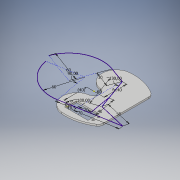
# Autodesk Inventor part: wstepna_geometria_wersja_2
Saved by Autodesk Inventor 2019 (Build 230136000, 136)
## iProperties
Created: 2022-02-09
Part Number: wstepna_geometria_wersja_2
Material: Generic
Document SubType Name: Modeling
Designer: Tomasz Krakowski
Density: 1 g/cm^3
Appearance: Default
Author: Tomasz Krakowski
Autodesk Inventor part; units mm, degrees
ref_plane "YZ Plane" through (0, 0, 0) normal (1, 0, 0) x (0, 1, 0)
ref_plane "XZ Plane" through (0, 0, 0) normal (0, 1, 0) x (-1, 0, 0)
ref_plane "XY Plane" through (0, 0, 0) normal (0, 0, 1) x (1, 0, 0)
sketch "Sketch1" plane through (0, 0, 0) normal (0, 1, 0) x (-1, 0, 0)
  arc A0 (-1.4142, 9.8995) -> (-10, 0) centre (0, 0) ccw
  line L0 (-39.5, 50) -> (0.5, 50)
  line L1 (0.5, 50) -> (0.5, 30)
  line L2 (0.5, 30) -> (-39.5, 30)
  line L3 (-39.5, 30) -> (-39.5, 50)
  line L4 (-39.5, 50) -> (0.5, 30) construction
  line L5 (0.5, 50) -> (-39.5, 30) construction
  line L6 (-10, 40) -> (-19.5, 40) construction
  circle A1 centre (4.5, 35.25) radius 1.9
  circle A2 centre (4.5, 44.75) radius 1.9
  line L7 (4.5, 44.75) -> (4.5, 35.25) construction
  circle A3 centre (-43.5, 44.75) radius 1.9
  circle A4 centre (-43.5, 35.25) radius 1.9
  line L8 (-43.5, 44.75) -> (-43.5, 35.25) construction
  line L9 (-43.5, 40) -> (-19.5, 40) construction
  line L10 (-10, 40) -> (4.5, 40) construction
  line L11 (-43.5, 44.75) -> (4.5, 44.75) construction
  line L12 (-43.5, 35.25) -> (4.5, 35.25) construction
  line L13 (-19.5, 40) -> (-19.5, 44.75) construction
  circle A5 centre (-10, 40) radius 9.75 construction
  circle A6 centre (-29, 40) radius 9.75 construction
  arc A7 (-2.7044, 60.2512) -> (-52.4397, 48.5007) centre (-10, -20) ccw
  arc A8 (-1.4142, 9.8995) -> (-2.7044, 60.2512) centre (-5, 35) ccw
  line L14 (-57.1731, 40) -> (-57.1731, 0)
  line L15 (-57.1731, 0) -> (0, 0) construction
  arc A9 (-52.4397, 48.5007) -> (-57.1731, 40) centre (-47.1731, 40) ccw
  line L16 (0, 0) -> (10, 0) construction
  line L17 (-10, 0) -> (-57.1731, 0) construction
  arc A10 (-10, 0) -> (-1.4142, -9.8995) centre (0, 0) ccw
  arc A11 (-52.4397, -48.5007) -> (-2.7044, -60.2512) centre (-10, 20) ccw
  arc A12 (-2.7044, -60.2512) -> (-1.4142, -9.8995) centre (-5, -35) ccw
  line L18 (-57.1731, -40) -> (-57.1731, 0)
  arc A13 (-57.1731, -40) -> (-52.4397, -48.5007) centre (-47.1731, -40) ccw
  point P0 (-57.1731, 45.3313)
  dimension "d0" = 20
  dimension "d1" = 40
  dimension "d2" = 20
  dimension "d3" = 10.5
  dimension "d4" = 48
  dimension "d5" = 3.8
  dimension "d6" = 9.5
  dimension "d7" = 19.5
  dimension "d8" = 10
  dimension "d9" = 40
  dimension "d11" = 10.5
  dimension "d12" = 35
  dimension "d13" = 5
  dimension "d16" = 10
  dimension "d17" = 20
  dimension "d18" = 10
  dimension "d19" = 40
  constraints: 38 end point, 17 point on circle, 14 centre point, 7 symmetric about line, 5 horizontal, 5 midpoint, 4 equal radius, 4 perpendicular, 4 tangent, 3 coincident, 3 point on line, 2 collinear, 2 parallel, 2 vertical, 4 other
  measures "d0" diameter of A0
  measures "d1" distance between parallel lines of L3 L1
  measures "d2" distance between parallel lines of L0 L2
  measures "d3" distance from line of L1 L6.start
  measures "d4" distance between parallel lines of L8 L7
  measures "d5" diameter of A1
  measures "d6" distance of L7.end L7.start
  measures "d7" diameter of A5
  measures "d8" horizontal distance of point (0, 0) L6.start
  measures "d9" vertical distance of point (0, 0) L6.start
  measures "d11" distance from line of L3 A6.centre
  measures "d12" vertical distance of point (0, 0) A8.centre
  measures "d13" horizontal distance of point (0, 0) A8.centre
  measures "d16" radius of A9
  measures "d17" vertical distance of point (0, 0) A7.centre
  measures "d18" horizontal distance of point (0, 0) A7.centre
  measures "d19" distance of L14.start L14.end
extrude "Extrusion1" add sketch "Sketch1" along normal blind 3
sketch "Sketch2" plane through (0, 3, 0) normal (0, 1, 0) x (1, 0, 0)
  line L0 (10, -40) -> (78.9365, -27.8446)
  line L1 (10, -40) -> (-0.5, -40) construction
  line L2 (-0.5, -30) -> (-0.5, -50) construction
  line L3 (-0.5, -50) -> (-0.5, -30) construction
  line L4 (10, -40) -> (-19.5442, -45.2094)
  line L5 (29.6962, -36.527) -> (22.7502, 2.8653)
  arc A0 (-89.0516, 3.4601) -> (-19.5442, -45.2094) centre (-29.9631, 13.879) ccw
  line L6 (-19.5442, -45.2094) -> (-29.9631, 13.879) construction
  line L7 (-29.9631, 13.879) -> (-89.0516, 3.4601) construction
  line L8 (10, -40) -> (10, -30) construction
  line L9 (10, 40) -> (-18.1402, 50.3985)
  line L10 (10, -30) -> (10, 40) construction
  arc A1 (-18.1402, 50.3985) -> (-95.2176, 14.9151) centre (-38.9372, -5.8819) ccw
  line L11 (-38.9372, -5.8819) -> (-18.1402, 50.3985) construction
  line L12 (-38.9372, -5.8819) -> (-95.2176, 14.9151) construction
  line L13 (10, 40) -> (30.2449, -16.4814)
  line L14 (30.2449, -16.4814) -> (10, 40) construction
  line L15 (78.9365, -27.8446) -> (30.2449, -16.4814)
  point P0 (0, 0)
  dimension "d23" = 10.5
  dimension "d24" = 30
  dimension "d25" = 70
  dimension "d27" = 40
  dimension "d28" = 20
  dimension "d29" = 60
  dimension "d30" = 90
  dimension "d31" = 100
  dimension "d32" = 30
  dimension "d33" = 40
  dimension "d34" = 40
  dimension "d36" = 60
  dimension "d37" = 60
  dimension "d38" = 130
  dimension "d40" = 50
  constraints: 28 end point, 4 point on circle, 3 perpendicular, 2 centre point, 2 collinear, 2 tangent, 1 midpoint, 1 point on line, 1 vertical
  measures "d23" distance from line of L2 L0.start
  measures "d24" distance of L0.start L4.end
  measures "d25" distance of L0.start L0.end
  measures "d27" distance of L5.start L5.end
  measures "d28" distance of L5.start L0.start
  measures "d29" radius of A0
  measures "d30" angle of L7 L6
  measures "d31" angle of L8 L4
  measures "d32" distance of L9.start L9.end
  measures "d33" vertical distance of L9.start point (0, 0)
  measures "d34" vertical distance of point (0, 0) L1.end
  measures "d36" distance of L11.start L12.end
  measures "d37" distance of L9.start L13.end
  measures "d38" angle of L9 L13
  measures "d40" distance of L0.end L13.end
equation "\"d11\" = d3"
equation "\"d33\" = d34"
body "Solid1"
